Autodesk Inventor part; units mm, degrees
(part 3 of 3)
sketch "Эскиз33" plane through (0, 30, 0) normal (0, 1, 0) x (1, 0, 0)
  line L0 (67.8823, -42.4264) -> (63.6396, -46.669) projected
  line L1 (67.8823, -42.4264) -> (38.5624, -13.1066) projected
  line L2 (38.5624, -13.1066) -> (38.5624, 13.1066) projected
  line L3 (38.5624, 13.1066) -> (67.8823, 42.4264) projected
  line L4 (63.6396, 46.669) -> (67.8823, 42.4264) projected
  line L5 (63.6396, 46.669) -> (36.7696, 19.799) projected
  arc A0 (33.9411, 19.799) -> (36.7696, 19.799) centre (35.3553, 21.2132) ccw projected
  line L6 (33.9411, 19.799) -> (19.799, 33.9411) projected
  arc A1 (19.799, 36.7696) -> (19.799, 33.9411) centre (21.2132, 35.3553) ccw projected
  line L7 (19.799, 36.7696) -> (46.669, 63.6396) projected
  line L8 (42.4264, 67.8823) -> (46.669, 63.6396) projected
  line L9 (42.4264, 67.8823) -> (13.1066, 38.5624) projected
  line L10 (13.1066, 38.5624) -> (-13.1066, 38.5624) projected
  line L11 (-13.1066, 38.5624) -> (-42.4264, 67.8823) projected
  line L12 (-46.669, 63.6396) -> (-42.4264, 67.8823) projected
  line L13 (-46.669, 63.6396) -> (-19.799, 36.7696) projected
  arc A2 (-19.799, 33.9411) -> (-19.799, 36.7696) centre (-21.2132, 35.3553) ccw projected
  line L14 (-19.799, 33.9411) -> (-33.9411, 19.799) projected
  arc A3 (-36.7696, 19.799) -> (-33.9411, 19.799) centre (-35.3553, 21.2132) ccw projected
  line L15 (-36.7696, 19.799) -> (-63.6396, 46.669) projected
  line L16 (-67.8823, 42.4264) -> (-63.6396, 46.669) projected
  line L17 (-67.8823, 42.4264) -> (-38.5624, 13.1066) projected
  line L18 (-38.5624, 13.1066) -> (-38.5624, -13.1066) projected
  line L19 (-38.5624, -13.1066) -> (-67.8823, -42.4264) projected
  line L20 (-63.6396, -46.669) -> (-67.8823, -42.4264) projected
  line L21 (-63.6396, -46.669) -> (-36.7696, -19.799) projected
  arc A4 (-33.9411, -19.799) -> (-36.7696, -19.799) centre (-35.3553, -21.2132) ccw projected
  line L22 (-33.9411, -19.799) -> (-19.799, -33.9411) projected
  arc A5 (-19.799, -36.7696) -> (-19.799, -33.9411) centre (-21.2132, -35.3553) ccw projected
  line L23 (-19.799, -36.7696) -> (-46.669, -63.6396) projected
  line L24 (-42.4264, -67.8823) -> (-46.669, -63.6396) projected
  line L25 (-42.4264, -67.8823) -> (-13.1066, -38.5624) projected
  line L26 (-13.1066, -38.5624) -> (13.1066, -38.5624) projected
  line L27 (13.1066, -38.5624) -> (42.4264, -67.8823) projected
  line L28 (46.669, -63.6396) -> (42.4264, -67.8823) projected
  line L29 (46.669, -63.6396) -> (19.799, -36.7696) projected
  arc A6 (19.799, -33.9411) -> (19.799, -36.7696) centre (21.2132, -35.3553) ccw projected
  line L30 (19.799, -33.9411) -> (33.9411, -19.799) projected
  arc A7 (36.7696, -19.799) -> (33.9411, -19.799) centre (35.3553, -21.2132) ccw projected
  line L31 (36.7696, -19.799) -> (63.6396, -46.669) projected
  line L32 (-13.1066, -33.5624) -> (-33.5624, -13.1066) projected
  line L33 (-33.5624, -13.1066) -> (-33.5624, 13.1066) projected
  line L34 (-33.5624, 13.1066) -> (-13.1066, 33.5624) projected
  line L35 (-13.1066, 33.5624) -> (13.1066, 33.5624) projected
  line L36 (13.1066, 33.5624) -> (33.5624, 13.1066) projected
  line L37 (33.5624, 13.1066) -> (33.5624, -13.1066) projected
  line L38 (33.5624, -13.1066) -> (13.1066, -33.5624) projected
  line L39 (13.1066, -33.5624) -> (-13.1066, -33.5624) projected
  arc A8 (46.3155, -73.8927) -> (46.3155, -85.2064) centre (51.9723, -79.5495) ccw projected
  line L40 (46.3155, -85.2064) -> (48.6736, -87.5645) projected
  arc A9 (45.42, -94.668) -> (48.7014, -93.0224) centre (0, 0) ccw projected
  arc A10 (43.0355, -94.1655) -> (45.42, -94.668) centre (44.5548, -92.8648) ccw projected
  line L41 (43.0355, -94.1655) -> (18.3802, -65.3664) projected
  arc A11 (18.3802, -65.3664) -> (17.477, -64.7643) centre (16.8609, -66.6671) ccw projected
  line L42 (17.477, -64.7643) -> (0.6161, -59.3045) projected
  arc A12 (0.6161, -59.3045) -> (-0.6161, -59.3045) centre (0, -61.2072) ccw projected
  line L43 (-0.6161, -59.3045) -> (-17.477, -64.7643) projected
  arc A13 (-17.477, -64.7643) -> (-18.3802, -65.3664) centre (-16.8609, -66.6671) ccw projected
  line L44 (-18.3802, -65.3664) -> (-43.0355, -94.1655) projected
  arc A14 (-45.42, -94.668) -> (-43.0355, -94.1655) centre (-44.5548, -92.8648) ccw projected
  arc A15 (-48.7014, -93.0224) -> (-45.42, -94.668) centre (0, 0) ccw projected
  line L45 (-48.6736, -87.5645) -> (-46.3155, -85.2064) projected
  arc A16 (-46.3155, -85.2064) -> (-46.3155, -73.8927) centre (-51.9723, -79.5495) ccw projected
  line L46 (-46.3155, -73.8927) -> (-73.8927, -46.3155) projected
  arc A17 (-73.8927, -46.3155) -> (-85.2064, -46.3155) centre (-79.5495, -51.9723) ccw projected
  line L47 (-85.2064, -46.3155) -> (-87.5645, -48.6736) projected
  arc A18 (-92.5543, 49.5852) -> (-92.5543, -49.5852) centre (0, 0) ccw projected
  line L48 (-87.5645, 48.6736) -> (-85.2064, 46.3155) projected
  arc A19 (-85.2064, 46.3155) -> (-73.8927, 46.3155) centre (-79.5495, 51.9723) ccw projected
  line L49 (-73.8927, 46.3155) -> (-46.3155, 73.8927) projected
  arc A20 (-46.3155, 73.8927) -> (-46.3155, 85.2064) centre (-51.9723, 79.5495) ccw projected
  line L50 (-46.3155, 85.2064) -> (-48.6736, 87.5645) projected
  arc A21 (48.7014, 93.0224) -> (-48.7014, 93.0224) centre (0, 0) ccw projected
  line L51 (48.6736, 87.5645) -> (46.3155, 85.2064) projected
  arc A22 (46.3155, 85.2064) -> (46.3155, 73.8927) centre (51.9723, 79.5495) ccw projected
  line L52 (46.3155, 73.8927) -> (73.8927, 46.3155) projected
  arc A23 (73.8927, 46.3155) -> (85.2064, 46.3155) centre (79.5495, 51.9723) ccw projected
  line L53 (85.2064, 46.3155) -> (87.5645, 48.6736) projected
  arc A24 (92.5543, -49.5852) -> (92.5543, 49.5852) centre (0, 0) ccw projected
  line L54 (87.5645, -48.6736) -> (85.2064, -46.3155) projected
  arc A25 (85.2064, -46.3155) -> (73.8927, -46.3155) centre (79.5495, -51.9723) ccw projected
  line L55 (73.8927, -46.3155) -> (46.3155, -73.8927) projected
  line L56 (-36.7696, -19.799) -> (-63.6396, -46.669) projected
  line L57 (-63.6396, -46.669) -> (-46.669, -63.6396) projected
  line L58 (-46.669, -63.6396) -> (-19.799, -36.7696) projected
  arc A26 (-19.799, -36.7696) -> (-19.799, -33.9411) centre (-21.2132, -35.3553) ccw projected
  line L59 (-19.799, -33.9411) -> (-33.9411, -19.799) projected
  arc A27 (-33.9411, -19.799) -> (-36.7696, -19.799) centre (-35.3553, -21.2132) ccw projected
  line L60 (-91.2033, -35.8602) -> (-90.4123, -37.7305) projected
  arc A28 (-90.4123, -37.7305) -> (-87.156, -38.3657) centre (-88.5702, -36.9514) ccw projected
  line L61 (-87.156, -38.3657) -> (-83.085, -34.2947) projected
  arc A29 (-76.014, -34.2947) -> (-83.085, -34.2947) centre (-79.5495, -37.8302) ccw projected
  line L62 (-76.014, -34.2947) -> (-67.8823, -42.4264) projected
  line L63 (-67.8823, -42.4264) -> (-38.5624, -13.1066) projected
  line L64 (-38.5624, -13.1066) -> (-38.5624, 13.1066) projected
  line L65 (-38.5624, 13.1066) -> (-67.8823, 42.4264) projected
  line L66 (-67.8823, 42.4264) -> (-76.014, 34.2947) projected
  arc A30 (-83.085, 34.2947) -> (-76.014, 34.2947) centre (-79.5495, 37.8302) ccw projected
  line L67 (-83.085, 34.2947) -> (-87.156, 38.3657) projected
  arc A31 (-87.156, 38.3657) -> (-90.4123, 37.7305) centre (-88.5702, 36.9514) ccw projected
  line L68 (-90.4123, 37.7305) -> (-91.2033, 35.8602) projected
  arc A32 (-91.2033, 35.8602) -> (-91.2033, -35.8602) centre (0, 0) ccw projected
  line L69 (-19.799, 36.7696) -> (-46.669, 63.6396) projected
  line L70 (-46.669, 63.6396) -> (-63.6396, 46.669) projected
  line L71 (-63.6396, 46.669) -> (-36.7696, 19.799) projected
  arc A33 (-36.7696, 19.799) -> (-33.9411, 19.799) centre (-35.3553, 21.2132) ccw projected
  line L72 (-33.9411, 19.799) -> (-19.799, 33.9411) projected
  arc A34 (-19.799, 33.9411) -> (-19.799, 36.7696) centre (-21.2132, 35.3553) ccw projected
  line L73 (34.2947, 83.085) -> (38.3657, 87.156) projected
  arc A35 (38.3657, 87.156) -> (37.7305, 90.4123) centre (36.9514, 88.5702) ccw projected
  line L74 (37.7305, 90.4123) -> (35.8602, 91.2033) projected
  arc A36 (35.8602, 91.2033) -> (-35.8602, 91.2033) centre (0, 0) ccw projected
  line L75 (-35.8602, 91.2033) -> (-37.7305, 90.4123) projected
  arc A37 (-37.7305, 90.4123) -> (-38.3657, 87.156) centre (-36.9514, 88.5702) ccw projected
  line L76 (-38.3657, 87.156) -> (-34.2947, 83.085) projected
  arc A38 (-34.2947, 76.014) -> (-34.2947, 83.085) centre (-37.8302, 79.5495) ccw projected
  line L77 (-34.2947, 76.014) -> (-42.4264, 67.8823) projected
  line L78 (-42.4264, 67.8823) -> (-13.1066, 38.5624) projected
  line L79 (-13.1066, 38.5624) -> (13.1066, 38.5624) projected
  line L80 (13.1066, 38.5624) -> (42.4264, 67.8823) projected
  line L81 (42.4264, 67.8823) -> (34.2947, 76.014) projected
  arc A39 (34.2947, 83.085) -> (34.2947, 76.014) centre (37.8302, 79.5495) ccw projected
  line L82 (36.7696, 19.799) -> (63.6396, 46.669) projected
  line L83 (63.6396, 46.669) -> (46.669, 63.6396) projected
  line L84 (46.669, 63.6396) -> (19.799, 36.7696) projected
  arc A40 (19.799, 36.7696) -> (19.799, 33.9411) centre (21.2132, 35.3553) ccw projected
  line L85 (19.799, 33.9411) -> (33.9411, 19.799) projected
  arc A41 (33.9411, 19.799) -> (36.7696, 19.799) centre (35.3553, 21.2132) ccw projected
  line L86 (83.085, -34.2947) -> (87.156, -38.3657) projected
  arc A42 (87.156, -38.3657) -> (90.4123, -37.7305) centre (88.5702, -36.9514) ccw projected
  line L87 (90.4123, -37.7305) -> (91.2033, -35.8602) projected
  arc A43 (91.2033, -35.8602) -> (91.2033, 35.8602) centre (0, 0) ccw projected
  line L88 (91.2033, 35.8602) -> (90.4123, 37.7305) projected
  arc A44 (90.4123, 37.7305) -> (87.156, 38.3657) centre (88.5702, 36.9514) ccw projected
  line L89 (87.156, 38.3657) -> (83.085, 34.2947) projected
  arc A45 (76.014, 34.2947) -> (83.085, 34.2947) centre (79.5495, 37.8302) ccw projected
  line L90 (76.014, 34.2947) -> (67.8823, 42.4264) projected
  line L91 (67.8823, 42.4264) -> (38.5624, 13.1066) projected
  line L92 (38.5624, 13.1066) -> (38.5624, -13.1066) projected
  line L93 (38.5624, -13.1066) -> (67.8823, -42.4264) projected
  line L94 (67.8823, -42.4264) -> (76.014, -34.2947) projected
  arc A46 (83.085, -34.2947) -> (76.014, -34.2947) centre (79.5495, -37.8302) ccw projected
  line L95 (63.6396, -46.669) -> (36.7696, -19.799) projected
  arc A47 (36.7696, -19.799) -> (33.9411, -19.799) centre (35.3553, -21.2132) ccw projected
  line L96 (33.9411, -19.799) -> (19.799, -33.9411) projected
  arc A48 (19.799, -33.9411) -> (19.799, -36.7696) centre (21.2132, -35.3553) ccw projected
  line L97 (19.799, -36.7696) -> (46.669, -63.6396) projected
  line L98 (46.669, -63.6396) -> (63.6396, -46.669) projected
  circle A49 centre (20.5578, -60.8546) radius 1.55 projected
  circle A50 centre (-20.5578, -60.8546) radius 1.55 projected
  line L99 (-33.5624, -13.1066) -> (-13.1066, -33.5624) projected
  line L100 (-13.1066, -33.5624) -> (13.1066, -33.5624) projected
  line L101 (13.1066, -33.5624) -> (33.5624, -13.1066) projected
  line L102 (33.5624, -13.1066) -> (33.5624, 13.1066) projected
  line L103 (33.5624, 13.1066) -> (13.1066, 33.5624) projected
  line L104 (13.1066, 33.5624) -> (-13.1066, 33.5624) projected
  line L105 (-13.1066, 33.5624) -> (-33.5624, 13.1066) projected
  line L106 (-33.5624, 13.1066) -> (-33.5624, -13.1066) projected
  line L107 (13.1066, -38.5624) -> (-13.1066, -38.5624) projected
  line L108 (-13.1066, -38.5624) -> (-42.4264, -67.8823) projected
  line L109 (-42.4264, -67.8823) -> (-37.1244, -73.1843) projected
  arc A51 (-37.1244, -73.1843) -> (-34.1909, -73.0707) centre (-35.7102, -71.7701) ccw projected
  line L110 (-34.1909, -73.0707) -> (-25.4187, -62.8242) projected
  arc A52 (-25.4187, -62.8242) -> (-24.842, -61.8893) centre (-28.1154, -60.5155) ccw projected
  line L111 (-24.842, -61.8893) -> (-23.8313, -59.4808) projected
  arc A53 (-21.0049, -57.3328) -> (-23.8313, -59.4808) centre (-20.5578, -60.8546) ccw projected
  line L112 (-21.0049, -57.3328) -> (-15.1585, -56.5907) projected
  arc A54 (-15.1585, -56.5907) -> (-14.5119, -56.4463) centre (-15.6055, -53.069) ccw projected
  line L113 (-14.5119, -56.4463) -> (-0.6161, -51.9466) projected
  arc A55 (0.6161, -51.9466) -> (-0.6161, -51.9466) centre (0, -53.8493) ccw projected
  line L114 (0.6161, -51.9466) -> (14.5119, -56.4463) projected
  arc A56 (14.5119, -56.4463) -> (15.1585, -56.5907) centre (15.6055, -53.069) ccw projected
  line L115 (15.1585, -56.5907) -> (21.0049, -57.3328) projected
  arc A57 (23.8313, -59.4808) -> (21.0049, -57.3328) centre (20.5578, -60.8546) ccw projected
  line L116 (23.8313, -59.4808) -> (24.842, -61.8893) projected
  arc A58 (24.842, -61.8893) -> (25.4187, -62.8242) centre (28.1154, -60.5155) ccw projected
  line L117 (25.4187, -62.8242) -> (34.1909, -73.0707) projected
  arc A59 (34.1909, -73.0707) -> (37.1244, -73.1843) centre (35.7102, -71.7701) ccw projected
  line L118 (37.1244, -73.1843) -> (42.4264, -67.8823) projected
  line L119 (42.4264, -67.8823) -> (13.1066, -38.5624) projected
  line L120 (-18.0817, 23.3345) -> (17.9183, 23.3345)
  line L121 (17.9183, 23.3345) -> (17.9183, -21.6655)
  line L122 (17.9183, -21.6655) -> (-18.0817, -21.6655) construction
  line L123 (-18.0817, -21.6655) -> (-18.0817, 23.3345)
  dimension "d331" = 36
  dimension "d332" = 45
  constraints: 8 end point, 2 parallel, 1 horizontal, 1 perpendicular, 8 other
  measures "d331" distance of L121.end L122.end
  measures "d332" distance of L120.end L121.end
extrude "Выдавливание23" add sketch "upper_frame" along normal blind 2 contours L0 S1 A32 S3 L47 A24 L46 A22 L45 S2 A23 A49 L87 A42 L37 A16 L38 A45 L86 A48 A19 S4 L50 A26 L55 A21 L42 S5 A36 S7 L61 A35 L101 A59 L98 S6 A10 S0 L3 A8 L1 A0 | L8 L10 A5 L16 A4 L20 L21 A31 L17 A15 L11 | A15 L17 L136 A87 L147 A98 L151 A94 L145 A31 L144 A93 L143 A30 L59 L142 A92 L150 A100 L148 A91 L141 A17 L139 A95 L138 A18 L67 L140 A90 L149 A85 L131 A81 L124 A3 L122 A83 L123 A29 L32 L125 A82 L130 A96 L146 A88 L137 A14 L135 A89 L134 | A14 L32 A29 L23 L100 L22 A12 L31 A13 L26 L24 | L79 L77 L78 A27 L60 A38 L70 L71 A17 L59 A30 | A3 L67 A18 L81 L84 L85 A39 L62 A28 L82 L83
sketch "Эскиз34" plane through (0, 32, 0) normal (0, 1, 0) x (1, 0, 0)
  point P0 (0, 0)
ref_plane "РабПлоскость12" through (0, 32, 0) normal (0, 1, 0) x (1, 0, 0)
sketch "Эскиз35" plane through (0, 32, 0) normal (0, 1, 0) x (1, 0, 0)
  circle A0 centre (0, 0) radius 18.0116
  circle A1 centre (0, 0) radius 23.1109
  constraints: 2 centre point, 2 coincident
extrude "Выдавливание24" add sketch "Эскиз35" along normal blind 25
sketch "Эскиз36" plane through (0, 57, 0) normal (0, 1, 0) x (1, 0, 0)
  circle A0 centre (0, 0) radius 45
  line L0 (-44.7, -4) -> (-41.9, -4)
  line L1 (-41.9, -4) -> (-41.9, 4)
  line L2 (-41.9, 4) -> (-44.7, 4)
  line L3 (-44.7, 4) -> (-44.7, -4)
  line L4 (0, 0) -> (-66.9557, 0) construction
  line L5 (-43.3, -4) -> (-43.3, 4) construction
  circle A1 centre (-43.3, -4) radius 0.75 construction
  circle A2 centre (-43.3, 0) radius 0.75 construction
  circle A3 centre (-43.3, 4) radius 0.75 construction
  line L6 (-40.3145, -12.0974) -> (-41.8753, -4.2511)
  line L7 (-43.0607, -12.6437) -> (-40.3145, -12.0974)
  line L8 (-44.6215, -4.7974) -> (-43.0607, -12.6437)
  line L9 (-41.8753, -4.2511) -> (-44.6215, -4.7974)
  line L10 (-37.1798, -19.73) -> (-40.2413, -12.3389)
  line L11 (-39.7667, -20.8015) -> (-37.1798, -19.73)
  line L12 (-42.8281, -13.4104) -> (-39.7667, -20.8015)
  line L13 (-40.2413, -12.3389) -> (-42.8281, -13.4104)
  line L14 (-32.6163, -26.6043) -> (-37.0609, -19.9525)
  line L15 (-34.9444, -28.1599) -> (-32.6163, -26.6043)
  line L16 (-39.389, -21.5081) -> (-34.9444, -28.1599)
  line L17 (-37.0609, -19.9525) -> (-39.389, -21.5081)
  line L18 (-26.7993, -32.4562) -> (-32.4562, -26.7993)
  line L19 (-28.7792, -34.4361) -> (-26.7993, -32.4562)
  line L20 (-34.4361, -28.7792) -> (-28.7792, -34.4361)
  line L21 (-32.4562, -26.7993) -> (-34.4361, -28.7792)
  line L22 (-19.9525, -37.0609) -> (-26.6043, -32.6163)
  line L23 (-21.5081, -39.389) -> (-19.9525, -37.0609)
  line L24 (-28.1599, -34.9444) -> (-21.5081, -39.389)
  line L25 (-26.6043, -32.6163) -> (-28.1599, -34.9444)
  line L26 (-12.3389, -40.2413) -> (-19.73, -37.1798)
  line L27 (-13.4104, -42.8281) -> (-12.3389, -40.2413)
  line L28 (-20.8015, -39.7667) -> (-13.4104, -42.8281)
  line L29 (-19.73, -37.1798) -> (-20.8015, -39.7667)
  line L30 (-4.2511, -41.8753) -> (-12.0974, -40.3145)
  line L31 (-4.7974, -44.6215) -> (-4.2511, -41.8753)
  line L32 (-12.6437, -43.0607) -> (-4.7974, -44.6215)
  line L33 (-12.0974, -40.3145) -> (-12.6437, -43.0607)
  line L34 (4, -41.9) -> (-4, -41.9)
  line L35 (4, -44.7) -> (4, -41.9)
  line L36 (-4, -44.7) -> (4, -44.7)
  line L37 (-4, -41.9) -> (-4, -44.7)
  line L38 (12.0974, -40.3145) -> (4.2511, -41.8753)
  line L39 (12.6437, -43.0607) -> (12.0974, -40.3145)
  line L40 (4.7974, -44.6215) -> (12.6437, -43.0607)
  line L41 (4.2511, -41.8753) -> (4.7974, -44.6215)
  line L42 (19.73, -37.1798) -> (12.3389, -40.2413)
  line L43 (20.8015, -39.7667) -> (19.73, -37.1798)
  line L44 (13.4104, -42.8281) -> (20.8015, -39.7667)
  line L45 (12.3389, -40.2413) -> (13.4104, -42.8281)
  line L46 (26.6043, -32.6163) -> (19.9525, -37.0609)
  line L47 (28.1599, -34.9444) -> (26.6043, -32.6163)
  line L48 (21.5081, -39.389) -> (28.1599, -34.9444)
  line L49 (19.9525, -37.0609) -> (21.5081, -39.389)
  line L50 (32.4562, -26.7993) -> (26.7993, -32.4562)
  line L51 (34.4361, -28.7792) -> (32.4562, -26.7993)
  line L52 (28.7792, -34.4361) -> (34.4361, -28.7792)
  line L53 (26.7993, -32.4562) -> (28.7792, -34.4361)
  line L54 (37.0609, -19.9525) -> (32.6163, -26.6043)
  line L55 (39.389, -21.5081) -> (37.0609, -19.9525)
  line L56 (34.9444, -28.1599) -> (39.389, -21.5081)
  line L57 (32.6163, -26.6043) -> (34.9444, -28.1599)
  line L58 (40.2413, -12.3389) -> (37.1798, -19.73)
  line L59 (42.8281, -13.4104) -> (40.2413, -12.3389)
  line L60 (39.7667, -20.8015) -> (42.8281, -13.4104)
  line L61 (37.1798, -19.73) -> (39.7667, -20.8015)
  line L62 (41.8753, -4.2511) -> (40.3145, -12.0974)
  line L63 (44.6215, -4.7974) -> (41.8753, -4.2511)
  line L64 (43.0607, -12.6437) -> (44.6215, -4.7974)
  line L65 (40.3145, -12.0974) -> (43.0607, -12.6437)
  line L66 (41.9, 4) -> (41.9, -4)
  line L67 (44.7, 4) -> (41.9, 4)
  line L68 (44.7, -4) -> (44.7, 4)
  line L69 (41.9, -4) -> (44.7, -4)
  line L70 (40.3145, 12.0974) -> (41.8753, 4.2511)
  line L71 (43.0607, 12.6437) -> (40.3145, 12.0974)
  line L72 (44.6215, 4.7974) -> (43.0607, 12.6437)
  line L73 (41.8753, 4.2511) -> (44.6215, 4.7974)
  line L74 (37.1798, 19.73) -> (40.2413, 12.3389)
  line L75 (39.7667, 20.8015) -> (37.1798, 19.73)
  line L76 (42.8281, 13.4104) -> (39.7667, 20.8015)
  line L77 (40.2413, 12.3389) -> (42.8281, 13.4104)
  line L78 (32.6163, 26.6043) -> (37.0609, 19.9525)
  line L79 (34.9444, 28.1599) -> (32.6163, 26.6043)
  line L80 (39.389, 21.5081) -> (34.9444, 28.1599)
  line L81 (37.0609, 19.9525) -> (39.389, 21.5081)
  line L82 (26.7993, 32.4562) -> (32.4562, 26.7993)
  line L83 (28.7792, 34.4361) -> (26.7993, 32.4562)
  line L84 (34.4361, 28.7792) -> (28.7792, 34.4361)
  line L85 (32.4562, 26.7993) -> (34.4361, 28.7792)
  line L86 (19.9525, 37.0609) -> (26.6043, 32.6163)
  line L87 (21.5081, 39.389) -> (19.9525, 37.0609)
  line L88 (28.1599, 34.9444) -> (21.5081, 39.389)
  line L89 (26.6043, 32.6163) -> (28.1599, 34.9444)
  line L90 (12.3389, 40.2413) -> (19.73, 37.1798)
  line L91 (13.4104, 42.8281) -> (12.3389, 40.2413)
  line L92 (20.8015, 39.7667) -> (13.4104, 42.8281)
  line L93 (19.73, 37.1798) -> (20.8015, 39.7667)
  line L94 (4.2511, 41.8753) -> (12.0974, 40.3145)
  line L95 (4.7974, 44.6215) -> (4.2511, 41.8753)
  line L96 (12.6437, 43.0607) -> (4.7974, 44.6215)
  line L97 (12.0974, 40.3145) -> (12.6437, 43.0607)
  line L98 (-4, 41.9) -> (4, 41.9)
  line L99 (-4, 44.7) -> (-4, 41.9)
  line L100 (4, 44.7) -> (-4, 44.7)
  line L101 (4, 41.9) -> (4, 44.7)
  line L102 (-12.0974, 40.3145) -> (-4.2511, 41.8753)
  line L103 (-12.6437, 43.0607) -> (-12.0974, 40.3145)
  line L104 (-4.7974, 44.6215) -> (-12.6437, 43.0607)
  line L105 (-4.2511, 41.8753) -> (-4.7974, 44.6215)
  line L106 (-19.73, 37.1798) -> (-12.3389, 40.2413)
  line L107 (-20.8015, 39.7667) -> (-19.73, 37.1798)
  line L108 (-13.4104, 42.8281) -> (-20.8015, 39.7667)
  line L109 (-12.3389, 40.2413) -> (-13.4104, 42.8281)
  line L110 (-26.6043, 32.6163) -> (-19.9525, 37.0609)
  line L111 (-28.1599, 34.9444) -> (-26.6043, 32.6163)
  line L112 (-21.5081, 39.389) -> (-28.1599, 34.9444)
  line L113 (-19.9525, 37.0609) -> (-21.5081, 39.389)
  line L114 (-32.4562, 26.7993) -> (-26.7993, 32.4562)
  line L115 (-34.4361, 28.7792) -> (-32.4562, 26.7993)
  line L116 (-28.7792, 34.4361) -> (-34.4361, 28.7792)
  line L117 (-26.7993, 32.4562) -> (-28.7792, 34.4361)
  line L118 (-37.0609, 19.9525) -> (-32.6163, 26.6043)
  line L119 (-39.389, 21.5081) -> (-37.0609, 19.9525)
  line L120 (-34.9444, 28.1599) -> (-39.389, 21.5081)
  line L121 (-32.6163, 26.6043) -> (-34.9444, 28.1599)
  line L122 (-40.2413, 12.3389) -> (-37.1798, 19.73)
  line L123 (-42.8281, 13.4104) -> (-40.2413, 12.3389)
  line L124 (-39.7667, 20.8015) -> (-42.8281, 13.4104)
  line L125 (-37.1798, 19.73) -> (-39.7667, 20.8015)
  line L126 (-41.8753, 4.2511) -> (-40.3145, 12.0974)
  line L127 (-44.6215, 4.7974) -> (-41.8753, 4.2511)
  line L128 (-43.0607, 12.6437) -> (-44.6215, 4.7974)
  line L129 (-40.3145, 12.0974) -> (-43.0607, 12.6437)
  circle A4 centre (0, 0) radius 18.0116
  point P0 (-44.7, 0)
  point P1 (-41.9, 0)
  point P2 (-45, 0)
  point P3 (-41.0949, -8.1743)
  point P4 (-41.6876, -12.3706)
  point P5 (-43.8411, -8.7205)
  point P6 (-43.2484, -4.5243)
  point P7 (-38.7106, -16.0344)
  point P8 (-38.4733, -20.2657)
  point P9 (-41.2974, -17.1059)
  point P10 (-41.5347, -12.8747)
  point P11 (-34.8386, -23.2784)
  point P12 (-33.7804, -27.3821)
  point P13 (-37.1667, -24.834)
  point P14 (-38.2249, -20.7303)
  point P15 (-29.6278, -29.6278)
  point P16 (-27.7893, -33.4462)
  point P17 (-31.6077, -31.6077)
  point P18 (-33.4462, -27.7893)
  point P19 (-23.2784, -34.8386)
  point P20 (-20.7303, -38.2249)
  point P21 (-24.834, -37.1667)
  point P22 (-27.3821, -33.7804)
  point P23 (-16.0344, -38.7106)
  point P24 (-12.8747, -41.5347)
  point P25 (-17.1059, -41.2974)
  point P26 (-20.2657, -38.4733)
  point P27 (-8.1743, -41.0949)
  point P28 (-4.5243, -43.2484)
  point P29 (-8.7205, -43.8411)
  point P30 (-12.3706, -41.6876)
  point P31 (0, -41.9)
  point P32 (4, -43.3)
  point P33 (0, -44.7)
  point P34 (-4, -43.3)
  point P35 (8.1743, -41.0949)
  point P36 (12.3706, -41.6876)
  point P37 (8.7205, -43.8411)
  point P38 (4.5243, -43.2484)
  point P39 (16.0344, -38.7106)
  point P40 (20.2657, -38.4733)
  point P41 (17.1059, -41.2974)
  point P42 (12.8747, -41.5347)
  point P43 (23.2784, -34.8386)
  point P44 (27.3821, -33.7804)
  point P45 (24.834, -37.1667)
  point P46 (20.7303, -38.2249)
  point P47 (29.6278, -29.6278)
  point P48 (33.4462, -27.7893)
  point P49 (31.6077, -31.6077)
  point P50 (27.7893, -33.4462)
  point P51 (34.8386, -23.2784)
  point P52 (38.2249, -20.7303)
  point P53 (37.1667, -24.834)
  point P54 (33.7804, -27.3821)
  point P55 (38.7106, -16.0344)
  point P56 (41.5347, -12.8747)
  point P57 (41.2974, -17.1059)
  point P58 (38.4733, -20.2657)
  point P59 (41.0949, -8.1743)
  point P60 (43.2484, -4.5243)
  point P61 (43.8411, -8.7205)
  point P62 (41.6876, -12.3706)
  point P63 (41.9, 0)
  point P64 (43.3, 4)
  point P65 (44.7, 0)
  point P66 (43.3, -4)
  point P67 (41.0949, 8.1743)
  point P68 (41.6876, 12.3706)
  point P69 (43.8411, 8.7205)
  point P70 (43.2484, 4.5243)
  point P71 (38.7106, 16.0344)
  point P72 (38.4733, 20.2657)
  point P73 (41.2974, 17.1059)
  point P74 (41.5347, 12.8747)
  point P75 (34.8386, 23.2784)
  point P76 (33.7804, 27.3821)
  point P77 (37.1667, 24.834)
  point P78 (38.2249, 20.7303)
  point P79 (29.6278, 29.6278)
  point P80 (27.7893, 33.4462)
  point P81 (31.6077, 31.6077)
  point P82 (33.4462, 27.7893)
  point P83 (23.2784, 34.8386)
  point P84 (20.7303, 38.2249)
  point P85 (24.834, 37.1667)
  point P86 (27.3821, 33.7804)
  point P87 (16.0344, 38.7106)
  point P88 (12.8747, 41.5347)
  point P89 (17.1059, 41.2974)
  point P90 (20.2657, 38.4733)
  point P91 (8.1743, 41.0949)
  point P92 (4.5243, 43.2484)
  point P93 (8.7205, 43.8411)
  point P94 (12.3706, 41.6876)
  point P95 (0, 41.9)
  point P96 (-4, 43.3)
  point P97 (0, 44.7)
  point P98 (4, 43.3)
  point P99 (-8.1743, 41.0949)
  point P100 (-12.3706, 41.6876)
  point P101 (-8.7205, 43.8411)
  point P102 (-4.5243, 43.2484)
  point P103 (-16.0344, 38.7106)
  point P104 (-20.2657, 38.4733)
  point P105 (-17.1059, 41.2974)
  point P106 (-12.8747, 41.5347)
  point P107 (-23.2784, 34.8386)
  point P108 (-27.3821, 33.7804)
  point P109 (-24.834, 37.1667)
  point P110 (-20.7303, 38.2249)
  point P111 (-29.6278, 29.6278)
  point P112 (-33.4462, 27.7893)
  point P113 (-31.6077, 31.6077)
  point P114 (-27.7893, 33.4462)
  point P115 (-34.8386, 23.2784)
  point P116 (-38.2249, 20.7303)
  point P117 (-37.1667, 24.834)
  point P118 (-33.7804, 27.3821)
  point P119 (-38.7106, 16.0344)
  point P120 (-41.5347, 12.8747)
  point P121 (-41.2974, 17.1059)
  point P122 (-38.4733, 20.2657)
  point P123 (-41.0949, 8.1743)
  point P124 (-43.2484, 4.5243)
  point P125 (-43.8411, 8.7205)
  point P126 (-41.6876, 12.3706)
  dimension "d346" = 90
  dimension "d347" = 2.8
  dimension "d348" = 8
  dimension "d350" = 1.7
  dimension "d351" = 1.5
  dimension "d352" = 1.5
  dimension "d353" = 1.5
  dimension "d356" = 360
  constraints: 260 end point, 5 midpoint, 4 centre point, 4 coincident, 2 horizontal, 2 parallel, 2 point on line, 1 horizontal alignment, 1 perpendicular, 387 other
  measures "d347" distance of L2.end L1.end
  measures "d348" distance of L1.end L0.end
  measures "d350" distance from line of point (-45, 0) L5
  measures "d351" diameter of A1
  measures "d352" diameter of A2
  measures "d353" diameter of A3
extrude "Выдавливание25" add sketch "Эскиз36" along normal blind 2
extrude "Выдавливание26" add sketch "Эскиз36" along normal blind 20 contours L19 L20 L21 L18
sketch "Эскиз37" plane through (-28.7792, 59, 34.4361) normal (-0.7071068, 0, 0.7071068) x (0.7071068, 0, 0.7071068)
  line L0 (-6, 17) -> (-2, 17)
  line L1 (-2, 17) -> (-2, 12)
  line L2 (-2, 12) -> (-6, 12)
  line L3 (-6, 12) -> (-6, 17)
  line L4 (-8, 18) -> (0, 18) projected
  line L5 (-4, -90.96) -> (-4, 36.16) projected
  point P0 (-4, -59)
  dimension "d362" = 4
  dimension "d363" = 5
  dimension "d364" = 1
  constraints: 8 end point, 2 parallel, 1 horizontal, 1 perpendicular, 1 other
  measures "d362" distance of L1.end L2.end
  measures "d363" distance of L0.end L1.end
  measures "d364" distance between parallel lines of L4 L0
extrude "Выдавливание27" add sketch "Эскиз37" along normal blind 2
pattern_circular "Круговой массив4" count 32 over 360 about axis through (0, -10, 0) along (0, 1, 0) of "Выдавливание26", "Выдавливание27"
sketch "Эскиз38" plane through (0, 59, 0) normal (0, 1, 0) x (1, 0, 0)
  line L0 (-8.5, -17.78) -> (35.95, -17.78)
  line L1 (35.95, -17.78) -> (35.95, 17.78)
  line L2 (35.95, 17.78) -> (-8.5, 17.78)
  line L3 (-8.5, 17.78) -> (-8.5, -17.78)
  line L4 (-8.5, 0) -> (35.95, 0) construction
  line L5 (13.725, -17.78) -> (13.725, 17.78) construction
  circle A0 centre (0, -15.24) radius 1.5 construction
  circle A1 centre (0, 15.24) radius 1.5 construction
  line L6 (0, -15.24) -> (0, 15.24) construction
  line L7 (-8.5, -8.5) -> (8.5, -8.5)
  line L8 (8.5, -8.5) -> (8.5, 8.5)
  line L9 (8.5, 8.5) -> (-8.5, 8.5)
  line L10 (-8.5, 8.5) -> (-8.5, -8.5) construction
  point P0 (0, 0)
  point P1 (-8.5, 0)
  point P2 (0, -8.5)
  point P3 (0, 0)
  dimension "d370" = 44.45
  dimension "d371" = 35.56
  dimension "d372" = 3
  dimension "d373" = 30.48
  dimension "d374" = 8.5
  dimension "d375" = 17
  dimension "d376" = 17
  constraints: 22 end point, 7 midpoint, 4 parallel, 2 centre point, 2 horizontal, 2 perpendicular, 2 point on line, 1 coincident, 1 symmetric about line, 1 vertical, 1 other
  measures "d370" distance of L2.end L1.end
  measures "d371" distance of L1.end L0.end
  measures "d372" diameter of A0
  measures "d373" distance of L6.start L6.end
  measures "d374" distance from line of L3 L6.start
  measures "d375" distance of L7.end L8.end
  measures "d376" distance of L8.end L9.end
extrude "Выдавливание28" add sketch "Эскиз38" along normal blind 1.6 contours L3 L7 L8 L9 L2 L1 L0
extrude "Выдавливание29" add sketch "Эскиз38" along normal blind 7.6 contours L3 L9 L8 L7
sketch "Эскиз39" plane through (0, 66.6, 0) normal (0, 1, 0) x (1, 0, 0)
  circle A0 centre (0, 0) radius 7.5
  dimension "d381" = 15
  constraints: 1 centre point, 1 coincident
  measures "d381" diameter of A0
extrude "Выдавливание30" add sketch "Эскиз39" along normal blind 7
sketch "Эскиз40" plane through (0, 59, 0) normal (0, 1, 0) x (1, 0, 0)
  circle A0 centre (-0.7467, 0) radius 22.5
  circle A1 centre (-0.7467, 0) radius 25.5
  point P0 (0, 0)
  dimension "d384" = 45
  dimension "d388" = 3
  constraints: 2 centre point, 1 coincident
  measures "d384" diameter of A0
  measures "d388" radial gap between concentric circles of A1 A0
ref_plane "РабПлоскость13" through (-0.7467, 109, 0) normal (0, 1, 0) x (1, 0, 0)
sketch "Эскиз41" plane through (-0.7467, 109, 0) normal (0, 1, 0) x (1, 0, 0)
  circle A0 centre (0, 0) radius 28.5
  point P0 (0.7467, 0)
  dimension "d389" = 57
  constraints: 1 centre point
  measures "d389" diameter of A0
extrude "Выдавливание32" add sketch "Эскиз41" along normal blind 4
extrude "Выдавливание33" add sketch "Эскиз40" along normal blind 14.6
